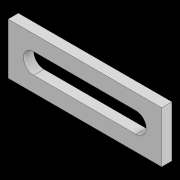
# Autodesk Inventor part: Platina Posterior Derecha
Saved by Autodesk Inventor 2021 (Build 250183000, 183)
## iProperties
Created: 2021-04-25
Part Number: Platina Posterior Derecha
Material: Generic
Document SubType Name: Modeling
Designer: maaro
Density: 1 g/cm^3
Appearance: Default
Author: maaro
Autodesk Inventor part; units mm, degrees
ref_plane "YZ Plane" through (0, 0, 0) normal (1, 0, 0) x (0, 1, 0)
ref_plane "XZ Plane" through (0, 0, 0) normal (0, 1, 0) x (-1, 0, 0)
ref_plane "XY Plane" through (0, 0, 0) normal (0, 0, 1) x (1, 0, 0)
sketch "Sketch1" plane through (0, 0, 0) normal (0, 0, 1) x (1, 0, 0)
  line L0 (-30, -10) -> (30, -10)
  line L1 (30, -10) -> (30, 10)
  line L2 (30, 10) -> (-30, 10)
  line L3 (-30, 10) -> (-30, -10)
  line L4 (-30, -10) -> (30, 10) construction
  line L5 (30, -10) -> (-30, 10) construction
  line L6 (-20, 0) -> (20, 0) construction
  line L7 (-20, -4) -> (20, -4)
  line L8 (20, 4) -> (-20, 4)
  arc A0 (-20, 4) -> (-20, -4) centre (-20, 0) ccw
  arc A1 (20, -4) -> (20, 4) centre (20, 0) ccw
  point P0 (0, 0)
  point P1 (0, 0)
  point P2 (0, 0)
  dimension "d0" = 60
  dimension "d1" = 20
  dimension "d2" = 8
  dimension "d3" = 40
  constraints: 20 end point, 4 midpoint, 4 point on circle, 4 tangent, 3 parallel, 2 centre point, 2 horizontal, 1 coincident, 1 perpendicular
  measures "d0" distance of L1.end L2.end
  measures "d1" distance of L0.end L1.end
  measures "d2" diameter of A1
  measures "d3" distance of L6.start L6.end
extrude "Extrusion1" add sketch "Sketch1" along normal mid plane 4
body "Solid1"
